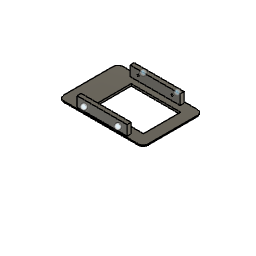
Enclosure-Back-With-Display-Cutout (Autodesk Fusion 360 design; units mm, degrees)
Autodesk Fusion 360 part; units mm, degrees
sketch "Sketch2" plane through (0, 0, -14.9563) normal (0, 0, -1) x (1, 0, 0)
  line L0 (77, -56) -> (3, -56)
  arc A0 (-1, -52) -> (3, -56) centre (3, -52) ccw
  line L1 (-1, -52) -> (-1, -3)
  arc A1 (3, 1) -> (-1, -3) centre (3, -3) ccw
  line L2 (3, 1) -> (77, 1)
  arc A2 (81, -3) -> (77, 1) centre (77, -3) ccw
  line L3 (81, -3) -> (81, -52)
  arc A3 (77, -56) -> (81, -52) centre (77, -52) ccw
  line L4 (77, 2.2) -> (3, 2.2)
  arc A4 (3, 2.2) -> (-2.2, -3) centre (3, -3) ccw
  line L5 (-2.2, -3) -> (-2.2, -52)
  arc A5 (-2.2, -52) -> (3, -57.2) centre (3, -52) ccw
  line L6 (3, -57.2) -> (77, -57.2)
  arc A6 (77, -57.2) -> (82.2, -52) centre (77, -52) ccw
  line L7 (82.2, -52) -> (82.2, -3)
  arc A7 (82.2, -3) -> (77, 2.2) centre (77, -3) ccw
  line L8 (20.4813, -48.1152) -> (20.4813, -7.1704) construction
  line L9 (15.4013, -48.5978) -> (15.4013, -44.229) construction
  line L10 (15.4013, -44.229) -> (13.5217, -44.229) construction
  line L11 (13.5217, -44.229) -> (13.5217, -49.1566) construction
  line L12 (13.5217, -49.1566) -> (73.8721, -49.1566) construction
  line L13 (73.8721, -49.1566) -> (73.8721, -6.5608) construction
  line L14 (73.8721, -6.5608) -> (13.5217, -6.5608) construction
  line L15 (13.5217, -6.5608) -> (13.5217, -16.0314) construction
  line L16 (13.5217, -16.0314) -> (15.4013, -16.0314) construction
  line L17 (15.4013, -16.0314) -> (15.4013, -7.1196) construction
  line L18 (15.4013, -7.1196) -> (73.3133, -7.1196) construction
  line L19 (73.3133, -7.1196) -> (73.3133, -48.5978) construction
  line L20 (73.3133, -48.5978) -> (15.4013, -48.5978) construction
  line L21 (21.8821, -9.4987) -> (21.8821, -46.2187) construction
  line L22 (21.8821, -46.2187) -> (70.8421, -46.2187) construction
  line L23 (70.8421, -46.2187) -> (70.8421, -9.4987) construction
  line L24 (70.8421, -9.4987) -> (21.8821, -9.4987) construction
  line L25 (21.6821, -46.4187) -> (71.0421, -46.4187)
  line L26 (71.0421, -46.4187) -> (71.0421, -9.2987)
  line L27 (71.0421, -9.2987) -> (21.6821, -9.2987)
  line L28 (21.6821, -9.2987) -> (21.6821, -46.4187)
  dimension "d20" = 0.2
extrude "Extrude1" add sketch "Sketch2" along normal blind 2 contours L0 A0 L1 A1 L2 A2 L3 A3 | L4 A4 L5 A5 L6 A6 L7 A7 makes body 1
sketch "Sketch3" plane through (0, 0, -14.9563) normal (0, 0, 1) x (-1, 0, 0)
  arc A0 (-77, 2.2) -> (-82.2, -3) centre (-77, -3) ccw
  line L0 (-82.2, -3) -> (-82.2, -52)
  arc A1 (-82.2, -52) -> (-77, -57.2) centre (-77, -52) ccw
  arc A2 (-3, -57.2) -> (2.2, -52) centre (-3, -52) ccw
  line L1 (2.2, -52) -> (2.2, -3)
  arc A3 (2.2, -3) -> (-3, 2.2) centre (-3, -3) ccw
  line L2 (-40, -59) -> (-40, 4) construction
  line L3 (-82.2, -27.5) -> (2.2, -27.5) construction
  line L4 (-3, 1) -> (-77, 1) construction
  line L5 (-77, -56) -> (-3, -56) construction
  line L6 (-15, 1) -> (-65, 1)
  line L7 (-65, 1) -> (-65, -3)
  line L8 (-65, -3) -> (-15, -3)
  line L9 (-15, -3) -> (-15, 1)
  line L10 (-15, -52) -> (-15, -56)
  line L11 (-15, -56) -> (-65, -56)
  line L12 (-65, -52) -> (-15, -52)
  line L13 (-65, -56) -> (-65, -52)
  dimension "d36" = 50
  dimension "d37" = 4
  dimension "d38" = 25
  constraint midpoint L0 L3.start
  constraint midpoint L1 L3.end
  constraint horizontal L6
  constraint vertical L7
  constraint horizontal L8
  constraint vertical L9
  constraint coincident L4.end L6
  constraint symmetric L3 L6.start L10.end
  constraint symmetric L3 L6.end L11.end
  constraint symmetric L3 L7.end L12.start
  constraint symmetric L3 L8.end L10.start
  measures "d36" distance of L6.start L6.end
  measures "d37" distance of L6.start L8.end
  measures "d38" distance of L2 L7
extrude "Extrude4" add sketch "Sketch3" along normal blind 10 separate body makes body 2 at (48.3333, 3, -11.6229) makes body 3 at (31.6667, 56, -8.2896)
fillet "Fillet1" radius 1 8 edges at (-2.2, 27.5, -16.9563) (-0.677, 55.677, -16.9563) (40, 57.2, -16.9563) (80.677, 55.677, -16.9563) (82.2, 27.5, -16.9563) (80.677, -0.677, -16.9563) (40, -2.2, -16.9563) (-0.677, -0.677, -16.9563) on bodies 1
sketch "sketch 1221" plane through (0, -2.2, 0) normal (0, -1, 0) x (1, 0, 0)
  circle A0 centre (23, -9.9563) radius 1
  circle A1 centre (57, -9.9563) radius 1
extrude "Extrude5" cut sketch "sketch 1221" against normal up to surface (5.2 mm away) bodies 2
sketch "sketch 1238" plane through (0, 57.2, 0) normal (0, 1, 0) x (-1, 0, 0)
  circle A0 centre (-57, -9.9563) radius 1
  circle A1 centre (-23, -9.9563) radius 1
extrude "Extrude6" cut sketch "sketch 1238" against normal up to surface (5.2 mm away) bodies 3
equation "d20 = margin"
equation "d21 = wall_thickness"
equation "d36 = lip_length"
equation "d37 = lip_width"
equation "d38 = lip_length / 2"
equation "d39 = lip_height"
equation "d45 = fillet_radius"
equation "margin = 0.2 mm"
equation "wall_thickness = 2 mm"
equation "lip_length = 50 mm"
equation "lip_width = 4 mm"
equation "lip_height = 10 mm"
equation "fillet_radius = 1 mm"
